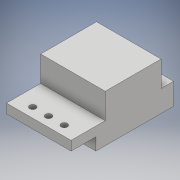
# Autodesk Inventor part: OKI-78SR
Saved by Autodesk Inventor 2018 (Build 220112000, 112)
## iProperties
Created: 2017-11-25
Part Number: OKI-78SR
Material: 一般
Document SubType Name: Modeling
Designer: sktom
Density: 1 g/cm^3
Appearance: 既定
Author: sktom
Autodesk Inventor part; units mm, degrees
ref_plane "YZ Plane" through (0, 0, 0) normal (1, 0, 0) x (0, 1, 0)
ref_plane "XZ Plane" through (0, 0, 0) normal (0, 1, 0) x (-1, 0, 0)
ref_plane "XY Plane" through (0, 0, 0) normal (0, 0, 1) x (1, 0, 0)
sketch "スケッチ1" plane through (0, 0, 0) normal (0, 0, 1) x (1, 0, 0)
  line L0 (-5.2, -8.25) -> (5.2, -8.25)
  line L1 (5.2, -8.25) -> (5.2, 8.25)
  line L2 (5.2, 8.25) -> (-5.2, 8.25)
  line L3 (-5.2, 8.25) -> (-5.2, -8.25)
  line L4 (-5.2, -8.25) -> (5.2, 8.25) construction
  line L5 (5.2, -8.25) -> (-5.2, 8.25) construction
  circle A0 centre (0, -6.68) radius 0.5
  circle A1 centre (2.54, -6.68) radius 0.5
  circle A2 centre (-2.54, -6.68) radius 0.5
  point P0 (0, 0)
  point P1 (0, 0)
  dimension "d0" = 10.4
  dimension "d1" = 16.5
  dimension "d2" = 1
  dimension "d3" = 2.54
  dimension "d4" = 2.54
  dimension "d5" = 1.57
  constraints: 12 end point, 3 centre point, 3 midpoint, 2 equal radius, 2 horizontal alignment, 2 parallel, 1 horizontal, 1 perpendicular, 1 vertical alignment
  measures "d0" distance of L1.end L2.end
  measures "d1" distance of L0.end L1.end
  measures "d2" diameter of A2
  measures "d3" distance of A0.centre A2.centre
  measures "d4" distance of A1.centre A0.centre
  measures "d5" distance from line of L0 A1.centre
extrude "押し出し1" add sketch "スケッチ1" along normal blind 1.5
sketch "スケッチ2" plane through (0, 0, 1.5) normal (0, 0, 1) x (1, 0, 0)
  line L0 (-5.2, 8.25) -> (-5.2, -8.25) projected
  line L1 (5.2, -8.25) -> (5.2, 8.25) projected
  line L2 (-5.2, 6.25) -> (5.2, 6.25)
  line L3 (5.2, 6.25) -> (5.2, -2.75)
  line L4 (5.2, -2.75) -> (-5.2, -2.75)
  line L5 (-5.2, -2.75) -> (-5.2, 6.25)
  line L6 (5.2, 8.25) -> (-5.2, 8.25) projected
  point P0 (0, 0)
  dimension "d8" = 2
  dimension "d9" = 9
  constraints: 8 end point, 2 parallel, 2 point on line, 1 horizontal, 1 perpendicular
  measures "d8" distance between parallel lines of L6 L2
  measures "d9" distance between parallel lines of L2 L4
extrude "押し出し2" add sketch "スケッチ2" along normal blind 4.1 contours L2 L1 L4 L0
sketch "スケッチ3" plane through (0, 0, 0) normal (0, 0, -1) x (-1, 0, 0)
  line L0 (-5.2, 8.25) -> (5.2, 8.25) projected
  line L1 (5.2, 8.25) -> (5.2, -8.25) projected
  line L2 (-5.2, 8.25) -> (5.2, 8.25)
  line L3 (5.2, 8.25) -> (5.2, -4.25)
  line L4 (5.2, -4.25) -> (-5.2, -4.25)
  line L5 (-5.2, -4.25) -> (-5.2, 8.25)
  line L6 (5.2, -8.25) -> (-5.2, -8.25) projected
  point P0 (0, 0)
  dimension "d12" = 4
  constraints: 8 end point, 2 parallel, 1 horizontal, 1 perpendicular, 1 point on line
  measures "d12" distance between parallel lines of L6 L4
extrude "押し出し3" add sketch "スケッチ3" along normal blind 2
